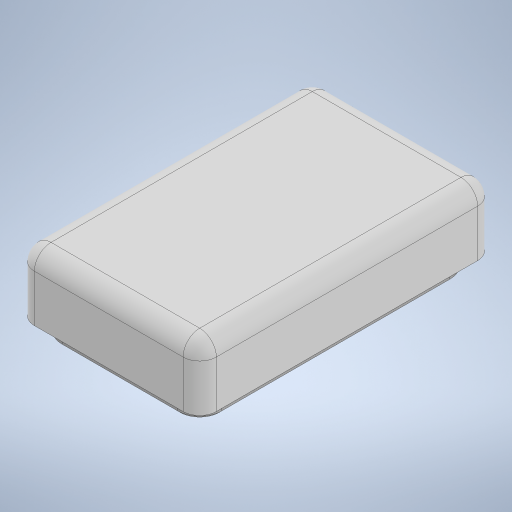
# Autodesk Inventor part: battery_housing_lid
Saved by Autodesk Inventor 2023.1 (Build 271208000, 208)
## iProperties
Created: 2026-04-28
Part Number: battery_housing_lid
Material: Generic
Document SubType Name: Modeling
Designer: Lars
Density: 1 g/cm^3
Appearance: Default
Author: Lars
Autodesk Inventor part; units mm, degrees
ref_plane "YZ Plane" through (0, 0, 0) normal (1, 0, 0) x (0, 1, 0)
ref_plane "XZ Plane" through (0, 0, 0) normal (0, 1, 0) x (-1, 0, 0)
ref_plane "XY Plane" through (0, 0, 0) normal (0, 0, 1) x (1, 0, 0)
sketch "Sketch1" plane through (0, 0, 0) normal (0, 1, 0) x (-1, 0, 0)
  line L0 (10.4, 23.55) -> (-10.4, 23.55)
  line L1 (-13.4, 20.55) -> (-13.4, -20.55)
  line L2 (-10.4, -23.55) -> (10.4, -23.55)
  line L3 (13.4, -20.55) -> (13.4, 20.55)
  line L4 (13.4, 23.55) -> (-13.4, -23.55) construction
  line L5 (-13.4, 23.55) -> (13.4, -23.55) construction
  arc A0 (13.4, 20.55) -> (10.4, 23.55) centre (10.4, 20.55) ccw
  arc A1 (10.4, -23.55) -> (13.4, -20.55) centre (10.4, -20.55) ccw
  arc A2 (-13.4, -20.55) -> (-10.4, -23.55) centre (-10.4, -20.55) ccw
  arc A3 (-10.4, 23.55) -> (-13.4, 20.55) centre (-10.4, 20.55) ccw
  line L6 (-10.4, 24.55) -> (10.4, 24.55)
  arc A4 (14.4, 20.55) -> (10.4, 24.55) centre (10.4, 20.55) ccw
  line L7 (14.4, 20.55) -> (14.4, -20.55)
  arc A5 (10.4, -24.55) -> (14.4, -20.55) centre (10.4, -20.55) ccw
  line L8 (10.4, -24.55) -> (-10.4, -24.55)
  arc A6 (-14.4, -20.55) -> (-10.4, -24.55) centre (-10.4, -20.55) ccw
  line L9 (-14.4, -20.55) -> (-14.4, 20.55)
  arc A7 (-10.4, 24.55) -> (-14.4, 20.55) centre (-10.4, 20.55) ccw
  line L10 (13.4, -26.55) -> (-13.4, -26.55)
  line L11 (-16.4, -23.55) -> (-16.4, 23.55)
  line L12 (-13.4, 26.55) -> (13.4, 26.55)
  line L13 (16.4, 23.55) -> (16.4, -23.55)
  line L14 (0, -26.55) -> (0, 26.55) construction
  line L15 (16.4, 0) -> (-16.4, 0) construction
  arc A8 (13.4, -26.55) -> (16.4, -23.55) centre (13.4, -23.55) ccw
  arc A9 (-16.4, -23.55) -> (-13.4, -26.55) centre (-13.4, -23.55) ccw
  arc A10 (-13.4, 26.55) -> (-16.4, 23.55) centre (-13.4, 23.55) ccw
  arc A11 (16.4, 23.55) -> (13.4, 26.55) centre (13.4, 23.55) ccw
  point P0 (0, 0)
  point P1 (16.4, -26.55)
  point P2 (-16.4, 26.55)
  point P3 (-16.4, -26.55)
  dimension "d0" = 26.8
  dimension "d1" = 47.1
  dimension "d2" = 3
  dimension "d4" = 1
  dimension "d23" = 53.1
  dimension "d24" = 32.8
  dimension "d25" = 3
  constraints: 32 end point, 24 point on circle, 16 tangent, 14 point on line, 12 centre point, 8 midpoint, 6 equal radius, 6 parallel, 3 perpendicular, 2 horizontal, 7 other
  measures "d0" distance of L5.end L4.end
  measures "d1" distance of L4.end L5.start
  measures "d2" radius of A0
  measures "d4" distance between parallel lines of L0 L6
  measures "d23" distance of point (-16.4, -26.55) point (-16.4, 26.55)
  measures "d24" distance of point (16.4, -26.55) point (-16.4, -26.55)
  measures "d25" radius of A8
extrude "Extrusion1" add sketch "Sketch1" against normal blind 2.9 contours L6 A4 L7 A5 L8 A6 L9 A7
extrude "Extrusion2" add sketch "Sketch1" along normal blind 8.5 contours L6 A4 L7 A5 L8 A6 L9 A7 | L10 A9 L11 A10 L12 A11 L13 A8
chamfer "Chamfer1" distance 0.5 angle 45 8 edges at (0, -2.9, 24.55) (-13.2284, -2.9, 23.3784) (-14.4, -2.9, 0) (-13.2284, -2.9, -23.3784) (0, -2.9, -24.55) (13.2284, -2.9, -23.3784) (14.4, -2.9, 0) (13.2284, -2.9, 23.3784)
sketch "Sketch2" plane through (0, 8.5, 0) normal (0, 1, 0) x (1, 0, 0)
  arc A0 (-13.4, -20.55) -> (-10.4, -23.55) centre (-10.4, -20.55) ccw projected
  line L0 (-13.4, -20.55) -> (-13.4, 20.55) projected
  arc A1 (-10.4, 23.55) -> (-13.4, 20.55) centre (-10.4, 20.55) ccw projected
  line L1 (-10.4, 23.55) -> (10.4, 23.55) projected
  arc A2 (13.4, 20.55) -> (10.4, 23.55) centre (10.4, 20.55) ccw projected
  line L2 (13.4, 20.55) -> (13.4, -20.55) projected
  arc A3 (10.4, -23.55) -> (13.4, -20.55) centre (10.4, -20.55) ccw projected
  line L3 (10.4, -23.55) -> (-10.4, -23.55) projected
  line L4 (-13.4, -26.55) -> (13.4, -26.55) projected
  arc A4 (13.4, -26.55) -> (16.4, -23.55) centre (13.4, -23.55) ccw projected
  line L5 (16.4, -23.55) -> (16.4, 23.55) projected
  arc A5 (16.4, 23.55) -> (13.4, 26.55) centre (13.4, 23.55) ccw projected
  line L6 (13.4, 26.55) -> (-13.4, 26.55) projected
  arc A6 (-13.4, 26.55) -> (-16.4, 23.55) centre (-13.4, 23.55) ccw projected
  line L7 (-16.4, 23.55) -> (-16.4, -23.55) projected
  arc A7 (-16.4, -23.55) -> (-13.4, -26.55) centre (-13.4, -23.55) ccw projected
  arc A8 (-13.4, -20.55) -> (-10.4, -23.55) centre (-10.4, -20.55) ccw projected
  line L8 (-13.4, -20.55) -> (-13.4, 20.55) projected
  arc A9 (-10.4, 23.55) -> (-13.4, 20.55) centre (-10.4, 20.55) ccw projected
  line L9 (-10.4, 23.55) -> (10.4, 23.55) projected
  arc A10 (13.4, 20.55) -> (10.4, 23.55) centre (10.4, 20.55) ccw projected
  line L10 (13.4, 20.55) -> (13.4, -20.55) projected
  arc A11 (10.4, -23.55) -> (13.4, -20.55) centre (10.4, -20.55) ccw projected
  line L11 (10.4, -23.55) -> (-10.4, -23.55) projected
  point P0 (0, 0)
extrude "Extrusion3" add sketch "Sketch2" along normal blind 3 contours L0 A1 L1 A2 L2 A3 L3 A0 | A7 L7 A6 L6 A5 L5 A4 L4
fillet "Fillet1" radius 3 16 edges at (12.5213, 8.5, 22.6713) (0, 8.5, 23.55) (-12.5213, 8.5, 22.6713) (-13.4, 8.5, 0) (-12.5213, 8.5, -22.6713) (0, 8.5, -23.55) (12.5213, 8.5, -22.6713) (13.4, 8.5, 0) (-15.5213, 11.5, -25.6713) (-16.4, 11.5, 0) (-15.5213, 11.5, 25.6713) (0, 11.5, 26.55) (15.5213, 11.5, 25.6713) (16.4, 11.5, 0) (15.5213, 11.5, -25.6713) (0, 11.5, -26.55)
sketch "Sketch3" plane through (-16.4, 0, -20.55) normal (-1, 0, 0) x (0, 0, 1)
  line L0 (0, 0) -> (0, 8.5) projected
  line L1 (41.1, 0) -> (41.1, 8.5) projected
  line L2 (4.9, 7) -> (35.3, 7)
  line L3 (38.8, 3.5) -> (38.8, 3.5)
  line L4 (35.3, 0) -> (4.9, 0)
  line L5 (1.4, 3.5) -> (1.4, 3.5)
  line L6 (1.4, 7) -> (38.8, 0) construction
  line L7 (38.8, 7) -> (1.4, 0) construction
  line L8 (-3, -2.9) -> (0, -2.9) projected
  line L9 (44.1, 5.5) -> (44.1, -2.9) projected
  line L10 (41.1, -2.9) -> (44.1, -2.9) projected
  line L11 (41.1, 8.5) -> (41.1, 5.5) projected
  line L12 (41.1, 5.5) -> (0, 5.5) construction
  line L13 (0, 5.5) -> (0, 8.5) projected
  line L14 (0, 8.5) -> (41.1, 8.5) projected
  line L15 (0, -2.9) -> (0, 5.5) projected
  line L16 (41.1, -2.4) -> (0, -2.4) projected
  line L17 (41.1, 0) -> (41.1, -2.4) projected
  line L18 (0, 0) -> (41.1, 0) projected
  line L19 (0, 0) -> (0, -2.4) projected
  arc A0 (4.9, 7) -> (1.4, 3.5) centre (4.9, 3.5) ccw
  arc A1 (38.8, 3.5) -> (35.3, 7) centre (35.3, 3.5) ccw
  arc A2 (35.3, 0) -> (38.8, 3.5) centre (35.3, 3.5) ccw
  arc A3 (1.4, 3.5) -> (4.9, 0) centre (4.9, 3.5) ccw
  line L20 (0, -2.9) -> (0, 5.5) projected
  line L21 (-3, -2.9) -> (-3, 5.5) projected
  line L22 (41.1, -2.9) -> (41.1, 5.5) projected
  line L23 (0, 5.5) -> (-3, 5.5) projected
  line L24 (44.1, 5.5) -> (41.1, 5.5) projected
  point P0 (20.55, 0)
  point P1 (20.1, 3.5)
  point P2 (20.55, 0)
  point P3 (1.4, 3.5)
  dimension "d15" = 37.4
  dimension "d16" = 7
  dimension "d19" = 5.3
  dimension "d20" = 3.5
  constraints: 12 end point, 9 point on line, 8 point on circle, 8 tangent, 4 centre point, 3 equal radius, 3 midpoint, 2 parallel, 1 horizontal, 1 perpendicular
  measures "d15" distance of L6.end L7.end
  measures "d16" distance of L7.start L6.end
  measures "d19" distance between parallel lines of L9 L3
  measures "d20" radius of A0
extrude "Extrusion4" cut sketch "Sketch3" against normal blind 6 contours A3 A0 L2 A1 A2 L4
equation "\"d20\" = 0.5 * d16"
body "Solid1"
